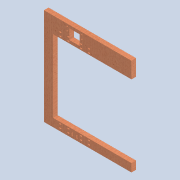
# Autodesk Inventor part: 0005-10-017 Batiu 2
Saved by Autodesk Inventor 2020 (Build 240168000, 168)
## iProperties
Created: 2020-12-18
Part Number: 0005-10-017 Batiu 2
Material: Wood (Maple)
Document SubType Name: Modeling
Designer: Iulian Bors
Density: 0.67 g/cm^3
Appearance: White Oak - Natural Medium Gloss
Mass: 666.639 g
Surface Area: 1589.64 cm^2
Volume: 994.984 cm^3
Author: Iulian Bors
Subject: 017
Autodesk Inventor part; units mm, degrees
ref_plane "YZ Plane" through (0, 0, 0) normal (1, 0, 0) x (0, 1, 0)
ref_plane "XZ Plane" through (0, 0, 0) normal (0, 1, 0) x (-1, 0, 0)
ref_plane "XY Plane" through (0, 0, 0) normal (0, 0, 1) x (1, 0, 0)
sketch "Sketch1" plane through (0, 0, 0) normal (0, 0, 1) x (1, 0, 0)
  line L0 (-190, 210) -> (190, 210)
  line L1 (190, 210) -> (190, -210)
  line L2 (190, -210) -> (-190, -210)
  line L3 (-190, -210) -> (-190, 210)
  point P0 (0, 0)
  point P1 (0, 210)
  point P2 (-190, 0)
  dimension "d0" = 380
  dimension "d1" = 420
  constraints: 8 end point, 2 midpoint, 2 parallel, 1 horizontal, 1 horizontal alignment, 1 perpendicular, 1 vertical alignment
  measures "d0" distance of L0.start L0.end
  measures "d1" distance of L2.end L0.start
extrude "Extrusion1" add sketch "Sketch1" along normal mid plane 20
sketch "Sketch5" plane through (0, 0, -10) normal (0, 0, -1) x (-1, 0, 0)
  line L0 (150, 140) -> (-190, 140)
  line L1 (-190, 140) -> (-190, -175)
  line L2 (-190, -175) -> (150, -175)
  line L3 (150, -175) -> (150, 140)
  line L4 (190, 210) -> (-190, 210) projected
  line L5 (-190, -210) -> (190, -210) projected
  line L6 (190, -210) -> (190, 210) projected
  point P0 (0, 0)
  dimension "d24" = 70
  dimension "d25" = 35
  dimension "d26" = 40
  constraints: 8 end point, 2 parallel, 1 horizontal, 1 perpendicular
  measures "d24" distance between parallel lines of L0 L4
  measures "d25" distance between parallel lines of L5 L2
  measures "d26" distance between parallel lines of L3 L6
extrude "Extrusion5" cut sketch "Sketch5" against normal through all
sketch "Sketch6" plane through (0, 0, -10) normal (0, 0, -1) x (-1, 0, 0)
  line L0 (66.806, -190) -> (66.806, -200) construction
  line L1 (64.556, -190) -> (64.556, -200)
  line L2 (69.056, -200) -> (69.056, -190)
  arc A0 (69.056, -190) -> (64.556, -190) centre (66.806, -190) ccw
  arc A1 (64.556, -200) -> (69.056, -200) centre (66.806, -200) ccw
  line L3 (-190, -210) -> (190, -210) projected
  line L4 (190, -210) -> (190, 210) projected
  line L5 (46.806, -190) -> (46.806, -200) construction
  line L6 (44.556, -190) -> (44.556, -200)
  line L7 (49.056, -200) -> (49.056, -190)
  arc A2 (49.056, -190) -> (44.556, -190) centre (46.806, -190) ccw
  arc A3 (44.556, -200) -> (49.056, -200) centre (46.806, -200) ccw
  point P0 (0, 0)
  point P1 (66.806, -195)
  point P2 (46.806, -195)
  dimension "d30" = 15
  dimension "d32" = 123.194
  dimension "d33" = 4.5
  dimension "d34" = 10
  dimension "d36" = 20
  constraints: 16 end point, 8 point on circle, 8 tangent, 4 centre point, 4 parallel, 2 midpoint, 2 vertical, 1 equal radius, 1 horizontal alignment
  measures "d30" distance from line of L3 point (66.806, -195)
  measures "d32" distance from line of L4 point (66.806, -195)
  measures "d33" distance between parallel lines of L1 L2
  measures "d34" distance of L0.start L0.end
  measures "d36" distance from line of L0 point (46.806, -195)
extrude "Extrusion6" cut sketch "Sketch6" against normal through all
sketch "Sketch8" plane through (0, 0, 10) normal (0, 0, 1) x (1, 0, 0)
  circle A0 centre (-57.306, 175) radius 2
  line L0 (-79.306, 153) -> (-35.306, 153)
  line L1 (-35.306, 153) -> (-35.306, 197)
  line L2 (-35.306, 197) -> (-79.306, 197)
  line L3 (-79.306, 197) -> (-79.306, 153)
  line L4 (-79.306, 153) -> (-35.306, 197) construction
  line L5 (-35.306, 153) -> (-79.306, 197) construction
  line L6 (190, 140) -> (190, 210) projected
  line L7 (-190, 210) -> (-190, -210) projected
  point P0 (0, 0)
  point P1 (-57.306, 175)
  point P2 (190, 175)
  dimension "d45" = 44
  dimension "d67" = 132.694
  constraints: 12 end point, 4 midpoint, 2 parallel, 2 perpendicular, 1 centre point, 1 horizontal, 1 horizontal alignment
  measures "d45" distance of L2.end L0.start
  measures "d67" distance from line of L7 A0.centre
extrude "Extrusion8" cut sketch "Sketch8" against normal through all contours A0 | L3 L2 L1 L0
sketch "Sketch9" plane through (0, 0, -10) normal (0, 0, -1) x (-1, 0, 0)
  line L0 (84.3, 163) -> (84.3, 147) construction
  line L1 (84.3, 147) -> (119.3, 147) construction
  line L2 (119.3, 147) -> (119.3, 163) construction
  line L3 (119.3, 163) -> (84.3, 163) construction
  line L4 (81.8, 163) -> (86.8, 163) construction
  line L5 (81.8, 160.75) -> (86.8, 160.75)
  line L6 (86.8, 165.25) -> (81.8, 165.25)
  arc A0 (81.8, 165.25) -> (81.8, 160.75) centre (81.8, 163) ccw
  arc A1 (86.8, 160.75) -> (86.8, 165.25) centre (86.8, 163) ccw
  line L7 (116.8, 163) -> (121.8, 163) construction
  line L8 (121.8, 147) -> (116.8, 147) construction
  line L9 (121.8, 149.25) -> (116.8, 149.25)
  line L10 (116.8, 144.75) -> (121.8, 144.75)
  arc A2 (121.8, 144.75) -> (121.8, 149.25) centre (121.8, 147) ccw
  arc A3 (116.8, 149.25) -> (116.8, 144.75) centre (116.8, 147) ccw
  line L11 (81.8, 147) -> (86.8, 147) construction
  line L12 (81.8, 144.75) -> (86.8, 144.75)
  line L13 (86.8, 149.25) -> (81.8, 149.25)
  arc A4 (81.8, 149.25) -> (81.8, 144.75) centre (81.8, 147) ccw
  arc A5 (86.8, 144.75) -> (86.8, 149.25) centre (86.8, 147) ccw
  circle A6 centre (121.306, 163) radius 2.75 projected
  line L14 (190, -210) -> (190, 210) projected
  line L15 (190, 210) -> (-190, 210) projected
  line L16 (116.8, 163) -> (121.8, 163) construction
  line L17 (116.8, 165.25) -> (121.8, 165.25)
  line L18 (121.8, 160.75) -> (116.8, 160.75)
  arc A7 (116.8, 165.25) -> (116.8, 160.75) centre (116.8, 163) ccw
  arc A8 (121.8, 160.75) -> (121.8, 165.25) centre (121.8, 163) ccw
  line L19 (-190, 210) -> (190, 210) projected
  line L20 (-190, 140) -> (150, 140) projected
  point P0 (0, 0)
  dimension "d50" = 35
  dimension "d51" = 16
  dimension "d52" = 5
  dimension "d53" = 4.5
  dimension "d54" = 68.694
  dimension "d55" = 47
  dimension "d56" = 70.7
  dimension "d68" = 7
  constraints: 44 end point, 16 point on circle, 16 tangent, 8 centre point, 6 parallel, 5 midpoint, 3 equal length, 3 equal radius, 2 perpendicular, 2 point on line, 1 coincident, 1 collinear
  measures "d50" distance of L3.start L3.end
  measures "d51" distance of L1.end L3.start
  measures "d52" distance of L4.start L4.end
  measures "d53" distance between parallel lines of L5 L6
  measures "d54" distance from line of A6.centre L14
  measures "d55" distance from line of A6.centre L15
  measures "d56" distance between parallel lines of L2 L14
  measures "d68" distance between parallel lines of L20 L1
extrude "Extrusion9" cut sketch "Sketch9" against normal through all contours A0 L6 A1 L5 | A2 L10 A3 L9 | A4 L13 A5 L12 | L17 A8 L18 A6 | A6 L18 A7 L17 picked at (120.7187, 163)
pattern_linear "Rectangular Pattern1" count 2 spacing 90 along (1, 0, 0) count 2 spacing 345 along (0, -1, 0) of "Extrusion9"
sketch "Sketch10" plane through (0, 0, -10) normal (0, 0, -1) x (-1, 0, 0)
  line L0 (89.306, 200) -> (25.306, 200) construction
  line L1 (25.306, 200) -> (25.306, 183) construction
  line L2 (25.306, 183) -> (89.306, 183) construction
  line L3 (89.306, 183) -> (89.306, 200) construction
  line L4 (35.306, 197) -> (79.306, 197) construction
  line L5 (190, 210) -> (-190, 210) construction
  point P0 (0, 0)
  point P1 (57.306, 200)
  point P2 (57.306, 197)
  dimension "d69" = 64
  dimension "d70" = 10
  dimension "d71" = 17
  constraints: 8 end point, 2 midpoint, 2 parallel, 1 horizontal, 1 perpendicular, 1 vertical alignment
  measures "d69" distance of L0.start L0.end
  measures "d70" distance between parallel lines of L5 L0
  measures "d71" distance of L2.end L0.start
hole "Hole1" at (-89.306, 183, -10) at (-89.306, 200, -10) at (-25.306, 200, -10) at (-25.306, 183, -10) direction (0, 0, 1) diameter 5 end through all
body "Solid1"
